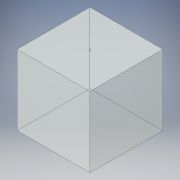
# Autodesk Inventor part: Workarea
Saved by Autodesk Inventor 2019.4 (Build 234330000, 330)
## iProperties
Created: 2019-12-12
Part Number: Workarea
Material: Generic
Document SubType Name: Modeling
Designer: Jorian Bruslind
Density: 1 g/cm^3
Appearance: Clear
Author: Jorian Bruslind
Autodesk Inventor part; units mm, degrees
ref_plane "YZ Plane" through (0, 0, 0) normal (1, 0, 0) x (0, 1, 0)
ref_plane "XZ Plane" through (0, 0, 0) normal (0, 1, 0) x (-1, 0, 0)
ref_plane "XY Plane" through (0, 0, 0) normal (0, 0, 1) x (1, 0, 0)
sketch "Sketch1" plane through (0, 0, 0) normal (0, 1, 0) x (-1, 0, 0)
  line L0 (0, 0) -> (276, 0)
  line L1 (276, 0) -> (276, -276)
  line L2 (276, -276) -> (0, -276)
  line L3 (0, -276) -> (0, 0)
  dimension "d0" = 276
  dimension "d1" = 276
  constraints: 8 end point, 2 parallel, 1 horizontal, 1 perpendicular
  measures "d0" distance of L1.end L2.end
  measures "d1" distance of L0.end L1.end
extrude "Extrusion1" add sketch "Sketch1" along normal blind 267
sketch "Sketch2" plane through (0, 267, 0) normal (0, 1, 0) x (1, 0, 0)
  line L0 (-276, 276) -> (-276, 0) projected
  line L1 (-276, 138) -> (-138, 138)
  line L2 (0, 276) -> (-276, 276) projected
  circle A0 centre (-138, 138) radius 2
  point P0 (0, 0)
  dimension "d4" = 4
  dimension "d5" = 138
  constraints: 2 end point, 1 centre point, 1 coincident, 1 midpoint, 1 parallel
  measures "d4" diameter of A0
  measures "d5" distance from line of L0 A0.centre
extrude "Extrusion2" cut sketch "Sketch2" against normal blind 5
body "Solid1"
